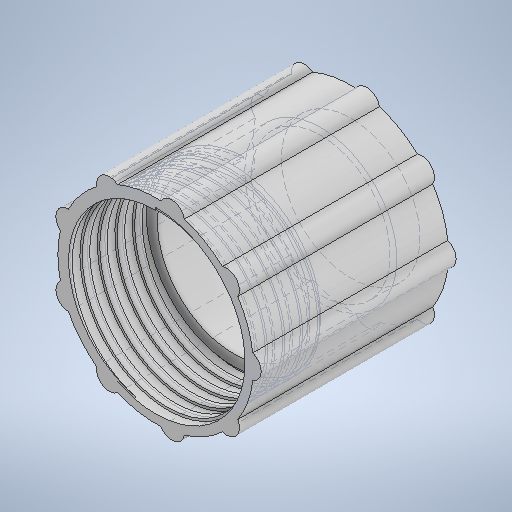
# Autodesk Inventor part: Red_Outer_Sleeve
Saved by Autodesk Inventor 2025.1 (Build 291241020, 241B)
## iProperties
Created: 2025-12-10
Part Number: Red_Outer_Sleeve
Material: Generic
Document SubType Name: Modeling
Designer: tapen
Density: 1 g/cm^3
Appearance: Default
Author: tapen
Autodesk Inventor part; units mm, degrees
ref_plane "YZ Plane" through (0, 0, 0) normal (1, 0, 0) x (0, 1, 0)
ref_plane "XZ Plane" through (0, 0, 0) normal (0, 1, 0) x (-1, 0, 0)
ref_plane "XY Plane" through (0, 0, 0) normal (0, 0, 1) x (1, 0, 0)
sketch "Sketch1" plane through (0, 0, 0) normal (0, 0, 1) x (1, 0, 0)
  point P0 (0, 0)
sketch "Sketch2" plane through (0, 0, 0) normal (0, 0, 1) x (1, 0, 0)
  circle A0 centre (0, 0) radius 12.715
  circle A1 centre (0, 0) radius 16.35
  arc A2 (16.2272, -2) -> (16.2272, 2) centre (15.4981, 0) ccw
  arc A3 (13.7163, 8.8986) -> (11.1452, 11.9627) centre (11.8723, 9.962) ccw
  arc A4 (4.7874, 15.6334) -> (0.8482, 16.328) centre (2.6912, 15.2627) ccw
  arc A5 (-6.3816, 15.0532) -> (-9.8457, 13.0532) centre (-7.7491, 13.4218) ccw
  arc A6 (-14.5646, 7.4294) -> (-15.9326, 3.6706) centre (-14.5635, 5.3007) ccw
  arc A7 (-15.9326, -3.6706) -> (-14.5646, -7.4294) centre (-14.5635, -5.3007) ccw
  arc A8 (-9.8457, -13.0532) -> (-6.3816, -15.0532) centre (-7.7491, -13.4218) ccw
  arc A9 (0.8482, -16.328) -> (4.7874, -15.6334) centre (2.6912, -15.2627) ccw
  arc A10 (11.1452, -11.9627) -> (13.7163, -8.8986) centre (11.8723, -9.962) ccw
  point P0 (13.7163, 8.8986)
  point P1 (4.7874, 15.6334)
  point P2 (0.8482, 16.328)
  point P3 (-6.3816, 15.0532)
  point P4 (-15.9326, 3.6706)
  point P5 (-15.9326, -3.6706)
  point P6 (-14.5646, -7.4294)
  point P7 (-6.3816, -15.0532)
  point P8 (0.8482, -16.328)
  point P9 (4.7874, -15.6334)
  point P10 (13.7163, -8.8986)
  dimension "d0" = 25.43
  dimension "d1" = 32.7
  dimension "d2" = 4
  dimension "d5" = 360
  constraints: 20 point on circle, 11 centre point, 2 coincident, 37 other
  measures "d0" diameter of A0
  measures "d1" diameter of A1
  measures "d2" distance of A1.end A1.start
extrude "Extrusion1" add sketch "Sketch2" along normal blind 32.6
sketch "Sketch3" plane through (0, 0, 0) normal (0, 0, -1) x (-1, 0, 0)
  circle A0 centre (0, 0) radius 11.585
  circle A1 centre (0, 0) radius 12.715
  dimension "d9" = 23.17
  constraints: 2 centre point, 2 coincident
  measures "d9" diameter of A0
extrude "Extrusion2" add sketch "Sketch3" against normal blind 5
sketch "Sketch4" plane through (0, 0, 32.6) normal (0, 0, 1) x (1, 0, 0)
  circle A0 centre (0, 0) radius 14.55
  dimension "d12" = 29.1
  constraints: 1 centre point, 1 coincident
  measures "d12" diameter of A0
extrude "Extrusion3" cut sketch "Sketch4" against normal blind 13
sketch "Sketch5" plane through (0, 0, 0) normal (1, 0, 0) x (0, 1, 0)
  line L0 (14.55, 32.6) -> (14.55, 19.6) projected
  line L1 (14.55, 32.5) -> (14.95, 32.5)
  line L2 (14.95, 32.5) -> (14.95, 34.17)
  line L3 (14.95, 34.17) -> (14.55, 34.17)
  line L4 (14.55, 34.17) -> (14.55, 32.5)
  line L5 (15.6334, 32.6) -> (11.9627, 32.6) projected
  line L6 (0, 0) -> (0, 48.4632) construction
  point P0 (14.75, 32.5)
  point P1 (14.75, 34.17)
  dimension "d15" = 0.4
  dimension "d16" = 1.67
  dimension "d18" = 1.57
  constraints: 10 end point, 2 midpoint, 2 parallel, 1 horizontal, 1 perpendicular, 1 point on line, 1 vertical
  measures "d15" distance of L3.end L2.end
  measures "d16" distance of L2.end L1.end
  measures "d18" distance from line of point (14.75, 34.17) L5
coil "Coil1" sketch "Sketch5" operation cut axis through (0, 0, 0) along (0, 0, -1) pitch 2.92 turns 5 hand right
body "Solid1"
